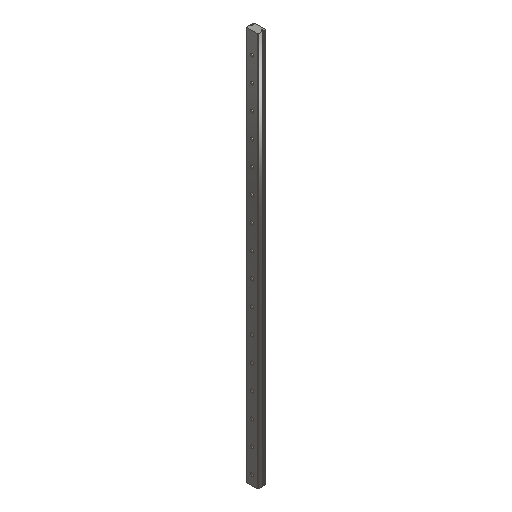
# Autodesk Inventor part: COTS_HIWIN_MGN12_RAIL_407mm
Saved by Autodesk Inventor 2026.1 (Build 301233000, 233)
## iProperties
Created: 2016-03-26
Part Number: COTS_HIWIN_MGN12_RAIL_407mm
Material: Ogólny
Document SubType Name: Modeling
Designer: Andrzej
Density: 1 g/cm^3
Appearance: Stal - polerowana
Mass: 34.6433 g
Surface Area: 195.927 cm^2
Volume: 34.6433 cm^3
Author: Andrzej
Autodesk Inventor part; units mm, degrees
ref_plane "YZ Plane" through (0, 0, 0) normal (1, 0, 0) x (0, 1, 0)
ref_plane "XZ Plane" through (0, 0, 0) normal (0, 1, 0) x (-1, 0, 0)
ref_plane "XY Plane" through (0, 0, 0) normal (0, 0, 1) x (1, 0, 0)
sketch "Szkic1" plane through (0, 0, 0) normal (0, 0, 1) x (1, 0, 0)
  line L0 (-0.5, 7.4119) -> (0, 8)
  line L1 (-0.5, 6.5901) -> (-0.5, 7.4119)
  arc A0 (0.0193, 6.0131) -> (-0.4182, 6.4505) centre (-0.9753, 5.4559) ccw
  arc A1 (-0.5, 6.5901) -> (-0.4182, 6.4505) centre (-0.34, 6.5901) ccw
  arc A2 (0.0193, 6.0131) -> (0.1589, 5.9313) centre (0.1589, 6.0913) ccw
  line L2 (0.5806, 5.9313) -> (0.1589, 5.9313)
  arc A3 (0.5806, 4.9806) -> (0.5806, 5.9313) centre (0.7358, 5.4559) ccw
  line L3 (0.1589, 4.9806) -> (0.5806, 4.9806)
  arc A4 (-0.4182, 4.4613) -> (0.0193, 4.8988) centre (-0.9753, 5.4559) ccw
  arc A5 (0.1589, 4.9806) -> (0.0193, 4.8988) centre (0.1589, 4.8206) ccw
  arc A6 (-0.4182, 4.4613) -> (-0.5, 4.3217) centre (-0.34, 4.3217) ccw
  line L4 (-0.5, 0.5) -> (-0.5, 4.3217)
  line L5 (0, 0) -> (-0.5, 0.5)
  line L6 (11, 0) -> (0, 0)
  line L7 (11.5, 0.5) -> (11, 0)
  line L8 (11.5, 4.3217) -> (11.5, 0.5)
  arc A7 (11.5, 4.3217) -> (11.4182, 4.4613) centre (11.34, 4.3217) ccw
  arc A8 (10.9807, 4.8988) -> (11.4182, 4.4613) centre (11.9753, 5.4559) ccw
  arc A9 (10.9807, 4.8988) -> (10.8411, 4.9806) centre (10.8411, 4.8206) ccw
  line L9 (10.4194, 4.9806) -> (10.8411, 4.9806)
  arc A10 (10.4194, 5.9313) -> (10.4194, 4.9806) centre (10.2642, 5.4559) ccw
  line L10 (10.8411, 5.9313) -> (10.4194, 5.9313)
  arc A11 (10.8411, 5.9313) -> (10.9807, 6.0131) centre (10.8411, 6.0913) ccw
  arc A12 (11.4182, 6.4505) -> (10.9807, 6.0131) centre (11.9753, 5.4559) ccw
  line L11 (11.5, 7.4119) -> (11.5, 6.5901)
  arc A13 (11.4182, 6.4505) -> (11.5, 6.5901) centre (11.34, 6.5901) ccw
  line L12 (11, 8) -> (11.5, 7.4119)
  line L13 (0, 8) -> (11, 8)
  constraints: 28 end point, 28 point on circle, 14 centre point
extrude "Wyciągnięcie proste1" add sketch "Szkic1" along normal blind 407
sketch "Szkic2" plane through (0, 8, 0) normal (0, 1, 0) x (1, 0, 0)
  line L0 (11, 0) -> (11, -407) projected
  line L1 (0, 0) -> (0, -407) projected
  line L2 (0, 0) -> (11, 0) projected
  line L3 (0, 0) -> (0, -407) projected
  line L4 (11, -407) -> (0, -407) projected
  line L5 (11, 0) -> (11, -407) projected
  point P0 (5.5, -10)
  point P1 (5.5, -35)
  point P2 (5.5, -60)
  point P3 (5.5, -85)
  point P4 (5.5, -110)
  point P5 (5.5, -135)
  point P6 (5.5, -160)
  point P7 (5.5, -185)
  point P8 (5.5, -210)
  point P9 (5.5, -235)
  point P10 (5.5, -260)
  point P11 (5.5, -285)
  point P12 (5.5, -310)
  point P13 (5.5, -335)
  point P14 (5.5, -360)
  point P15 (5.5, -385)
  dimension "d2" = 11
  dimension "d3" = 5.5
  dimension "d4" = 10
  dimension "d7" = 25
  constraints: 1 vertical, 15 other
  measures "d2" distance between parallel lines of L0 L1
  measures "d3" distance from line of L0 point (5.5, -10)
  measures "d4" distance from line of L2 point (5.5, -10)
  measures "d7" distance of point (5.5, -10) point (5.5, -35)
hole "Otwór1" at (5.5, 8, 10) at (5.5, 8, 35) at (5.5, 8, 60) at (5.5, 8, 85) at (5.5, 8, 110) at (5.5, 8, 135) at (5.5, 8, 160) at (5.5, 8, 185) at (5.5, 8, 210) at (5.5, 8, 235) at (5.5, 8, 260) at (5.5, 8, 285) at (5.5, 8, 310) at (5.5, 8, 335) at (5.5, 8, 360) at (5.5, 8, 385) direction (0, -1, 0) diameter 3.5 end through all
hole "Otwór2" at (5.5, 8, 210) at (5.5, 8, 385) at (5.5, 8, 360) at (5.5, 8, 335) at (5.5, 8, 310) at (5.5, 8, 285) at (5.5, 8, 260) at (5.5, 8, 235) at (5.5, 8, 185) at (5.5, 8, 160) at (5.5, 8, 135) at (5.5, 8, 110) at (5.5, 8, 85) at (5.5, 8, 60) at (5.5, 8, 35) at (5.5, 8, 10) direction (0, -1, 0) diameter 6 depth 4.6
